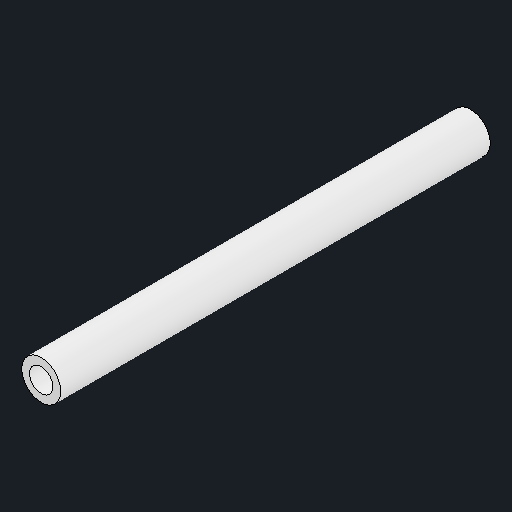
# Autodesk Inventor part: pihti-simulation-ceramic-sleeve-10x6x110
Saved by Autodesk Inventor 2027.1 (Build 311270010, 270A)
## iProperties
Created: 2024-05-16
Part Number: pihti-simulation-ceramic-sleeve-10x6x110
Material: Polystyrene
Document SubType Name: Modeling
Designer: kuzmin
Density: 1.021 g/cm^3
Appearance: Smooth - White
Description: Simulation simplification: continuous 10 mm OD, 6 mm bore, 110 mm ceramic sleeve replacing eleven stacked rings. Source material property requires simulation review.
Mass: 5.64532 g
Surface Area: 56.2973 cm^2
Volume: 5.5292 cm^3
Author: kuzmin
Autodesk Inventor part; units mm, degrees
ref_plane "YZ Plane" through (0, 0, 0) normal (1, 0, 0) x (0, 1, 0)
ref_plane "XZ Plane" through (0, 0, 0) normal (0, 1, 0) x (-1, 0, 0)
ref_plane "XY Plane" through (0, 0, 0) normal (0, 0, 1) x (1, 0, 0)
sketch "Sketch1" plane through (0, 0, 0) normal (0, 0, 1) x (1, 0, 0)
  circle A0 centre (0, 0) radius 3
  circle A1 centre (0, 0) radius 5
  dimension "d0" = 10
  dimension "d1" = 6
  constraints: 2 centre point, 2 coincident
  measures "d0" diameter of A1
  measures "d1" diameter of A0
extrude "Extrusion1" add sketch "Sketch1" along normal blind 110
body "Solid1"
